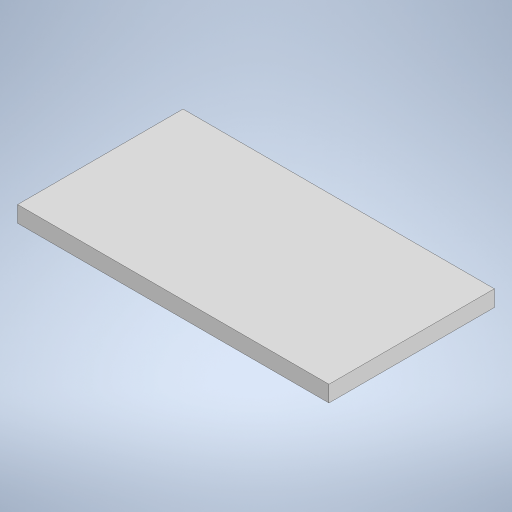
# Autodesk Inventor part: Battery Cover2.0
Saved by Autodesk Inventor 2023 (Build 270158000, 158)
## iProperties
Created: 2022-12-10
Part Number: Battery Cover2.0
Material: Generic
Document SubType Name: Modeling
Designer: spfow
Density: 1 g/cm^3
Appearance: Default
Author: spfow
Autodesk Inventor part; units mm, degrees
ref_plane "YZ Plane" through (0, 0, 0) normal (1, 0, 0) x (0, 1, 0)
ref_plane "XZ Plane" through (0, 0, 0) normal (0, 1, 0) x (-1, 0, 0)
ref_plane "XY Plane" through (0, 0, 0) normal (0, 0, 1) x (1, 0, 0)
sketch "Sketch1" plane through (0, 0, 0) normal (0, 1, 0) x (-1, 0, 0)
  line L0 (4.573, -187.8072) -> (65.533, -187.8072)
  line L1 (65.533, -187.8072) -> (65.533, -220.1922)
  line L2 (65.533, -220.1922) -> (4.573, -220.1922)
  line L3 (4.573, -220.1922) -> (4.573, -187.8072)
  point P0 (0, 0)
  dimension "d0" = 60.96
  dimension "d1" = 32.385
  constraints: 8 end point, 2 parallel, 1 horizontal, 1 perpendicular
  measures "d0" distance of L1.end L2.end
  measures "d1" distance of L0.end L1.end
extrude "Extrusion1" add sketch "Sketch1" along normal blind 3.175
body "Solid1"
